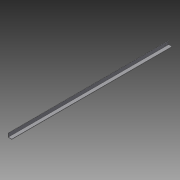
# Autodesk Inventor part: Y_Rail-SquareBar-Rev3
Saved by Autodesk Inventor 2015 (Build 190159000, 159)
## iProperties
Created: 2017-01-10
Part Number: Y_Rail-SquareBar-Rev3
Material: Generic
Document SubType Name: Modeling
Designer: Guy
Density: 1 g/cm^3
Appearance: Default
Author: Guy
Autodesk Inventor part; units mm, degrees
ref_plane "YZ Plane" through (0, 0, 0) normal (1, 0, 0) x (0, 1, 0)
ref_plane "XZ Plane" through (0, 0, 0) normal (0, 1, 0) x (-1, 0, 0)
ref_plane "XY Plane" through (0, 0, 0) normal (0, 0, 1) x (1, 0, 0)
sketch "Sketch1" plane through (0, 0, 0) normal (0, 0, 1) x (1, 0, 0)
  line L0 (0, 0) -> (0, 30)
  line L1 (0, 30) -> (3, 30)
  line L2 (3, 30) -> (3, 3)
  line L3 (3, 3) -> (30, 3)
  line L4 (30, 3) -> (30, 0)
  line L5 (30, 0) -> (0, 0)
  dimension "d0" = 30
  dimension "d1" = 30
  dimension "d2" = 3
  dimension "d3" = 3
  constraints: 12 end point, 5 perpendicular, 1 vertical
  measures "d0" distance between parallel lines of L0 L4
  measures "d1" distance between parallel lines of L5 L1
  measures "d2" distance between parallel lines of L0 L2
  measures "d3" distance between parallel lines of L5 L3
extrude "Extrusion1" add sketch "Sketch1" along normal blind 1300
sketch "Sketch2" plane through (3, 3, 0) normal (1, 0, 0) x (0, 0, -1)
  line L0 (0, 27) -> (0, 0) projected
  line L1 (0, 27) -> (-1300, 27) projected
  line L2 (-1300, 0) -> (-1300, 27) projected
  line L3 (0, 0) -> (-1300, 0) projected
  circle A0 centre (-8, 19) radius 2.5
  circle A1 centre (-8, 7) radius 2.5
  circle A2 centre (-28, 19) radius 2.5
  circle A3 centre (-28, 7) radius 2.5
  point P0 (0, -3)
  dimension "d6" = 5
  dimension "d7" = 5
  dimension "d8" = 5
  dimension "d9" = 5
  dimension "d10" = 8
  dimension "d11" = 8
  dimension "d12" = 20
  dimension "d13" = 20
  dimension "d14" = 8
  dimension "d15" = 8
  dimension "d16" = 12
  dimension "d17" = 12
  constraints: 4 centre point
  measures "d6" diameter of A0
  measures "d7" diameter of A1
  measures "d8" diameter of A2
  measures "d9" diameter of A3
  measures "d10" distance from line of A0.centre L1
  measures "d11" distance from line of A2.centre L1
  measures "d12" distance of A0.centre A2.centre
  measures "d13" distance of A1.centre A3.centre
  measures "d14" distance from line of L0 A0.centre
  measures "d15" distance from line of L0 A1.centre
  measures "d16" distance of A1.centre A0.centre
  measures "d17" distance of A3.centre A2.centre
extrude "Extrusion2" cut sketch "Sketch2" against normal blind 1300 contours A0 | A1 | A2 | A3
body "Solid1"
